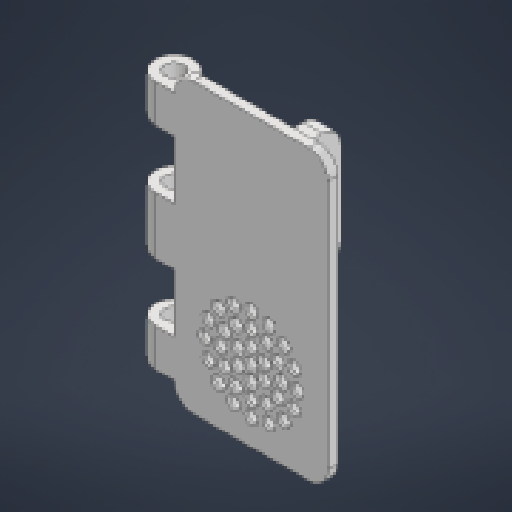
# Autodesk Inventor part: lid2
Saved by Autodesk Inventor 2026 (Build 300175050, 175E)
## iProperties
Created: 2025-05-28
Part Number: lid2
Material: Generic
Document SubType Name: Modeling
Designer: niall
Density: 1 g/cm^3
Appearance: Default
Author: niall
## iProperties of the stored document lid2_3DPrint.ipt
Created: 2025-05-28
Part Number: lid2_3DPrint
Material: Generic
Document SubType Name: Modeling
Designer: niall
Density: 1 g/cm^3
Appearance: Default
Author: niall
Autodesk Inventor part; units mm, degrees
ref_plane "YZ Plane" through (0, 0, 0) normal (1, 0, 0) x (0, 1, 0)
ref_plane "XZ Plane" through (0, 0, 0) normal (0, 1, 0) x (-1, 0, 0)
ref_plane "XY Plane" through (0, 0, 0) normal (0, 0, 1) x (1, 0, 0)
sketch "Sketch1" plane through (0, 0, 0) normal (0, 0, 1) x (1, 0, 0)
  arc A0 (30, -75) -> (40, -65) centre (30, -65) ccw projected
  line L0 (40, -65) -> (40, 65) projected
  arc A1 (40, 65) -> (30, 75) centre (30, 65) ccw projected
  line L1 (30, 75) -> (-30, 75) projected
  arc A2 (-30, 75) -> (-40, 65) centre (-30, 65) ccw projected
  line L2 (-40, 65) -> (-40, 42.5) projected
  arc A3 (-40, -65) -> (-30, -75) centre (-30, -65) ccw projected
  line L3 (-30, -75) -> (30, -75) projected
  line L4 (-30, 70) -> (30, 70) projected
  arc A4 (35, 65) -> (30, 70) centre (30, 65) ccw projected
  line L5 (35, 65) -> (35, -65) projected
  arc A5 (30, -70) -> (35, -65) centre (30, -65) ccw projected
  line L6 (30, -70) -> (-30, -70) projected
  arc A6 (-35, -65) -> (-30, -70) centre (-30, -65) ccw projected
  line L7 (-35, -65) -> (-35, 65) projected
  arc A7 (-30, 70) -> (-35, 65) centre (-30, 65) ccw projected
  line L8 (-40, 42.5) -> (-40, 17.5) projected
  line L9 (-40, 17.5) -> (-40, -17.5) projected
  line L10 (-40, -17.5) -> (-40, -42.5) projected
  line L11 (-40, -42.5) -> (-40, -65) projected
  point P0 (0, 0)
extrude "Extrusion1" add sketch "Sketch1" along normal blind 5 contours L3 A3 L11 L10 L9 L8 L2 A2 L1 A1 L0 A0 | L4 A4 L5 A5 L6 A6 L7 A7
sketch "Sketch4" plane through (0, 0, 0) normal (0, 0, -1) x (-1, 0, 0)
  arc A0 (35, 65) -> (30, 70) centre (30, 65) ccw projected
  line L0 (35, -65) -> (35, 65) projected
  arc A1 (30, -70) -> (35, -65) centre (30, -65) ccw projected
  line L1 (-30, -70) -> (30, -70) projected
  arc A2 (-35, -65) -> (-30, -70) centre (-30, -65) ccw projected
  line L2 (-35, 65) -> (-35, -65) projected
  arc A3 (-30, 70) -> (-35, 65) centre (-30, 65) ccw projected
  line L3 (30, 70) -> (-30, 70) projected
  line L4 (-35, 65) -> (-22, 65)
  line L5 (-22, 70) -> (-12, 70)
  line L6 (-12, 70) -> (-12, 60)
  line L7 (-12, 60) -> (-22, 60)
  line L8 (-22, 60) -> (-22, 70)
  line L9 (-12, 60) -> (-22, 60)
  line L10 (-22, 60) -> (-22, 17)
  line L11 (-22, 17) -> (-12, 17)
  line L12 (-12, 17) -> (-12, 60)
  line L13 (-12, 17) -> (-22, 17)
  line L14 (-22, 17) -> (-22, 7)
  line L15 (-22, 7) -> (-12, 7)
  line L16 (-12, 7) -> (-12, 17)
  point P0 (0, 0)
  dimension "d24" = 13
  dimension "d25" = 10
  dimension "d26" = 10
  dimension "d27" = 43
  dimension "d28" = 10
  constraints: 26 end point, 7 parallel, 3 horizontal, 3 perpendicular, 3 point on line
  measures "d24" distance of L2.start L4.end
  measures "d25" distance of L6.end L7.end
  measures "d26" distance of L5.end L6.end
  measures "d27" distance of L10.end L9.end
  measures "d28" distance of L14.end L13.end
extrude "Extrusion4" add sketch "Sketch4" along normal blind 20 contours L6 L7 L8 L3 | L12 L11 L10 L7 | L16 L15 L14 L11
sketch "Sketch5" plane through (12, 7, 0) normal (-1, 0, 0) x (0, 0, 1)
  line L0 (0, 63) -> (-10, 63)
  line L1 (-10, 63) -> (-10, 53)
  line L2 (-10, 53) -> (0, 53)
  line L3 (0, 53) -> (0, 63)
  line L4 (-10, 53) -> (0, 53)
  line L5 (0, 53) -> (0, 10)
  line L6 (0, 10) -> (-10, 10)
  line L7 (-10, 10) -> (-10, 53)
  point P0 (0, -7)
  dimension "d31" = 10
  dimension "d32" = 10
  dimension "d33" = 43
  constraints: 16 end point, 4 parallel, 2 horizontal, 2 perpendicular, 1 point on line
  measures "d31" distance of L2.end L1.end
  measures "d32" distance of L1.end L0.end
  measures "d33" distance of L4.end L5.end
extrude "Extrusion5" cut sketch "Sketch5" against normal up to surface (10 mm away) contours L5 L6 L7 L2
fillet "Fillet1" radius 10 2 edges at (17, 70, -20) (17, 7, -20)
fillet "Fillet2" radius 5 4 edges at (17, 60, 0) (17, 60, -10) (17, 17, 0) (17, 17, -10)
sketch "Sketch6" plane through (-40, -65, 0) normal (-1, 0, 0) x (0, 0, 1)
  line L0 (0, 130) -> (0, 0) projected
  line L1 (0, 0) -> (5, 0) projected
  line L2 (5, 130) -> (5, 0) projected
  line L3 (0, 130) -> (5, 130) projected
  line L4 (5, 130) -> (5, 140) projected
  line L5 (5, 130) -> (0, 130)
  line L6 (0, 130) -> (0, 110)
  line L7 (0, 110) -> (5, 110)
  line L8 (5, 110) -> (5, 130)
  line L9 (5, 0) -> (0, 0)
  line L10 (0, 0) -> (0, 20)
  line L11 (0, 20) -> (5, 20)
  line L12 (5, 20) -> (5, 0)
  line L13 (-5, 50) -> (5, 50)
  line L14 (5, 50) -> (5, 80)
  line L15 (5, 80) -> (-5, 80)
  line L16 (-5, 80) -> (-5, 50)
  line L17 (-5, 50) -> (5, 80) construction
  line L18 (5, 50) -> (-5, 80) construction
  line L19 (5, 130) -> (-15, 130)
  line L20 (-15, 130) -> (-15, 110)
  line L21 (-15, 110) -> (5, 110)
  line L22 (5, 110) -> (5, 130)
  line L23 (5, 80) -> (-15, 80)
  line L24 (-15, 80) -> (-15, 50)
  line L25 (-15, 50) -> (5, 50)
  line L26 (5, 50) -> (5, 80)
  line L27 (5, 20) -> (-15, 20)
  line L28 (-15, 20) -> (-15, 0)
  line L29 (-15, 0) -> (5, 0)
  line L30 (5, 0) -> (5, 20)
  point P0 (0, 65)
  point P1 (5, 50)
  dimension "d38" = 20
  dimension "d39" = 20
  dimension "d40" = 30
  dimension "d41" = 20
  dimension "d42" = 20
  dimension "d43" = 20
  dimension "d50" = 0
  constraints: 52 end point, 12 parallel, 6 horizontal, 6 perpendicular, 3 point on line, 2 midpoint
  measures "d38" distance of L6.end L5.end
  measures "d39" distance of L9.end L10.end
  measures "d40" distance of L14.end L13.end
  measures "d41" distance of L21.end L20.end
  measures "d42" distance of L25.end L24.end
  measures "d43" distance of L29.end L28.end
  measures "d50" distance between parallel lines of L13 L25
extrude "Extrusion6" add sketch "Sketch6" along normal blind 20 contours L3 L2 L7 L0 | L0 L21 L20 L19 | L15 L2 L13 L0 | L0 L13 L16 L15 | L16 L25 L24 L23 | L11 L2 L1 L0 | L0 L29 L28 L27
sketch "Sketch7" plane through (-40, 65, 0) normal (0, 1, 0) x (1, 0, 0)
  line L0 (0, -5) -> (-20, -5) projected
  line L1 (0, 15) -> (-20, 15) projected
  line L2 (0, -5) -> (-20, -5)
  line L3 (-20, -5) -> (-20, 15)
  line L4 (-20, 15) -> (0, 15)
  line L5 (0, 15) -> (0, -5)
  circle A0 centre (-10, 5) radius 5
  point P0 (40, 0)
  dimension "d46" = 10
  constraints: 8 end point, 2 parallel, 1 centre point, 1 horizontal, 1 perpendicular
  measures "d46" diameter of A0
extrude "Extrusion7" cut sketch "Sketch7" against normal up to surface (130 mm away) contours A0
fillet "Fillet3" radius 10 9 edges at (-60, 55, 5) (-60, 0, 5) (-60, 0, -15) (-60, -55, -15) (-60, -55, 5) (-40, -55, -15) (-40, 0, -15) (-40, 55, -15) (-60, 55, -15)
sketch "Sketch8" plane through (0, 0, 0) normal (0, 0, -1) x (-1, 0, 0)
  arc A0 (-40, -65) -> (-30, -75) centre (-30, -65) ccw projected
  line L0 (-40, -65) -> (-30, -65)
  line L1 (-30, -65) -> (-30, -75)
  line L2 (-30, -75) -> (-40, -75)
  line L3 (-40, -75) -> (-40, -65)
  line L4 (40, 15) -> (40, -15) projected
  line L5 (-40, -75) -> (40, -75)
  line L6 (40, -75) -> (40, 0)
  line L7 (40, 0) -> (-40, 0)
  line L8 (-40, 0) -> (-40, -75)
  line L9 (40, 0) -> (0, 0)
  line L10 (40, -37.5) -> (40, 0)
  circle A1 centre (0, -37.5) radius 2.5
  line L11 (0, -37.5) -> (0, -29.5)
  circle A2 centre (0, -29.5) radius 2.5
  line L12 (0, -29.5) -> (0, -21.5)
  circle A3 centre (0, -21.5) radius 2.5
  circle A4 centre (-6.9282, -33.5) radius 2.5
  circle A5 centre (-6.9282, -41.5) radius 2.5
  circle A6 centre (0, -45.5) radius 2.5
  circle A7 centre (6.9282, -41.5) radius 2.5
  circle A8 centre (6.9282, -33.5) radius 2.5
  circle A9 centre (-8, -23.6436) radius 2.5
  circle A10 centre (-13.8564, -29.5) radius 2.5
  circle A11 centre (-16, -37.5) radius 2.5
  circle A12 centre (-13.8564, -45.5) radius 2.5
  circle A13 centre (-8, -51.3564) radius 2.5
  circle A14 centre (0, -53.5) radius 2.5
  circle A15 centre (8, -51.3564) radius 2.5
  circle A16 centre (13.8564, -45.5) radius 2.5
  circle A17 centre (16, -37.5) radius 2.5
  circle A18 centre (13.8564, -29.5) radius 2.5
  circle A19 centre (8, -23.6436) radius 2.5
  line L13 (0, -21.5) -> (0, -13.5)
  circle A20 centre (0, -13.5) radius 2.5
  circle A21 centre (-9.1844, -15.3269) radius 2.5
  circle A22 centre (-16.9706, -20.5294) radius 2.5
  circle A23 centre (-22.1731, -28.3156) radius 2.5
  circle A24 centre (-24, -37.5) radius 2.5
  circle A25 centre (-22.1731, -46.6844) radius 2.5
  circle A26 centre (-16.9706, -54.4706) radius 2.5
  circle A27 centre (-9.1844, -59.6731) radius 2.5
  circle A28 centre (0, -61.5) radius 2.5
  circle A29 centre (9.1844, -59.6731) radius 2.5
  circle A30 centre (16.9706, -54.4706) radius 2.5
  circle A31 centre (22.1731, -46.6844) radius 2.5
  circle A32 centre (24, -37.5) radius 2.5
  circle A33 centre (22.1731, -28.3156) radius 2.5
  circle A34 centre (16.9706, -20.5294) radius 2.5
  circle A35 centre (9.1844, -15.3269) radius 2.5
  point P0 (0, 0)
  dimension "d51" = 5
  dimension "d52" = 8
  dimension "d53" = 5
  dimension "d54" = 8
  dimension "d55" = 5
  dimension "d58" = 360
  dimension "d62" = 360
  dimension "d64" = 8
  dimension "d65" = 5
  dimension "d68" = 360
  constraints: 35 centre point, 26 end point, 4 coincident, 4 parallel, 3 horizontal, 2 perpendicular, 1 midpoint, 1 vertical, 71 other
  measures "d51" diameter of A1
  measures "d52" distance of L11.start L11.end
  measures "d53" diameter of A2
  measures "d54" distance of L12.start L12.end
  measures "d55" diameter of A3
  measures "d64" distance of L13.start L13.end
  measures "d65" diameter of A20
extrude "Extrusion8" cut sketch "Sketch8" against normal up to surface (5 mm away) contours A1 | A2 L12 L11 | L11 L12 A2 | A3 L13 L12 | L12 L13 A3 | A4 | A5 | A6 | A7 | A8 | A9 | A10 | A11 | A12 | A13 | A14 | A15 | A16 | A17 | A18 | A19 | A20 | A21 | A22 | A23 | A24 | A25 | A26 | A27 | A28 | A29 | A30 | A31 | A32 | A33 | A34 | A35
fillet "Fillet4" radius 1 69 edges at (-11.3564, -45.5, 0) (-11.3564, -45.5, 5) (-21.5, -37.5, 0) (11.6844, -15.3269, 5) (2.5, -21.5, 5) (2.5, -21.5, 0) (10.5, -23.6436, 0) (10.5, -23.6436, 5) (-19.6731, -28.3156, 0) (-19.6731, -28.3156, 5) (16.3564, -29.5, 0) (16.3564, -29.5, 5) (-21.5, -37.5, 5) (-4.4282, -33.5, 0) (-4.4282, -33.5, 5) (26.5, -37.5, 5) (2.5, -61.5, 5) (2.5, -61.5, 0) (11.6844, -15.3269, 0) (10.5, -51.3564, 0) (10.5, -51.3564, 5) (2.5, -29.5, 0) (2.5, -37.5, 0) (2.5, -37.5, 5) (-4.4282, -41.5, 0) (-4.4282, -41.5, 5) (9.4282, -41.5, 0) (9.4282, -41.5, 5) (24.6731, -46.6844, 0) (24.6731, -46.6844, 5) (2.5, -53.5, 0) (2.5, -53.5, 5) (2.5, -29.5, 5) (-13.5, -37.5, 0) (-14.4706, -20.5294, 0) (-14.4706, -20.5294, 5) (-5.5, -23.6436, 0) (-5.5, -23.6436, 5) (24.6731, -28.3156, 0) (24.6731, -28.3156, 5) (16.3564, -45.5, 0) (16.3564, -45.5, 5) (-13.5, -37.5, 5) (2.5, -45.5, 0) (2.5, -45.5, 5) (-19.6731, -46.6844, 0) (-19.6731, -46.6844, 5) (11.6844, -59.6731, 0) (11.6844, -59.6731, 5) (-6.6844, -59.6731, 5) (-6.6844, -59.6731, 0) (2.5, -13.5, 0) (2.5, -13.5, 5) (-6.6844, -15.3269, 0) (-6.6844, -15.3269, 5) (19.4706, -20.5294, 0) (19.4706, -20.5294, 5) (9.4282, -33.5, 0) (9.4282, -33.5, 5) (18.5, -37.5, 0) (18.5, -37.5, 5) (-11.3564, -29.5, 5) (19.4706, -54.4706, 0) (19.4706, -54.4706, 5) (-5.5, -51.3564, 5) (-5.5, -51.3564, 0) (-14.4706, -54.4706, 0) (-11.3564, -29.5, 0) (-14.4706, -54.4706, 5)
equation "\"d70\" = d51"
body "Solid1"
